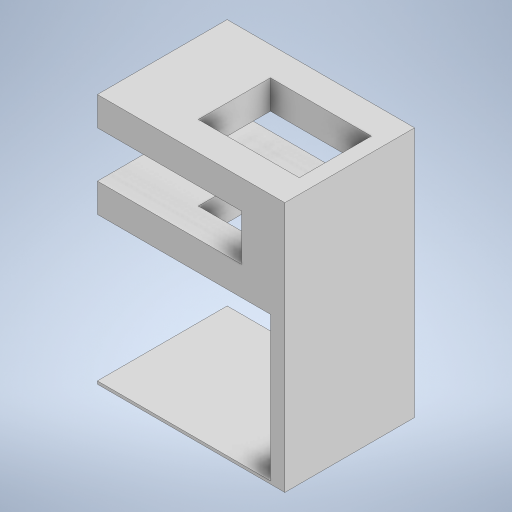
# Autodesk Inventor part: Стенка
Saved by Autodesk Inventor 2023 (Build 270158000, 158)
## iProperties
Created: 2022-04-28
Part Number: Стенка
Material: Типовые
Document SubType Name: Modeling
Designer: User
Density: 1 g/cm^3
Appearance: По умолчанию
Author: User
Autodesk Inventor part; units mm, degrees
ref_plane "YZ Plane" through (0, 0, 0) normal (1, 0, 0) x (0, 1, 0)
ref_plane "XZ Plane" through (0, 0, 0) normal (0, 1, 0) x (-1, 0, 0)
ref_plane "XY Plane" through (0, 0, 0) normal (0, 0, 1) x (1, 0, 0)
sketch "Эскиз1" plane through (0, 0, 0) normal (0, 1, 0) x (-1, 0, 0)
  line L0 (0, 0) -> (60, 0)
  line L1 (60, 0) -> (60, -45)
  line L2 (60, -45) -> (0, -45)
  line L3 (0, -45) -> (0, 0)
  line L4 (0, -22.5) -> (0, 0)
  line L5 (0, 0) -> (0, -10)
  line L6 (0, -10) -> (35, -10)
  line L7 (35, -10) -> (35, -35)
  line L8 (35, -35) -> (0, -35)
  line L9 (35, -22.5) -> (45, -22.5)
  dimension "d0" = 60
  dimension "d1" = 45
  dimension "d3" = 10
  dimension "d4" = 35
  dimension "d5" = 25
  dimension "d6" = 10
  constraints: 20 end point, 4 perpendicular, 2 horizontal, 2 midpoint, 2 parallel, 2 point on line, 1 collinear
  measures "d0" distance of L1.end L2.end
  measures "d1" distance of L0.end L1.end
  measures "d3" distance of L0.start L5.end
  measures "d4" distance of L5.end L6.end
  measures "d5" distance of L6.end L7.end
  measures "d6" distance of L9.start L9.end
extrude "Выдавливание1" add sketch "Эскиз1" along normal blind 10 contours L0 L1 L2 L3 L8 L7 L6
sketch "Эскиз3" plane through (0, 0, -35) normal (1, 0, 0) x (0, 0, -1)
  line L0 (10, 10) -> (-35, 10) projected
  line L1 (10, 10) -> (-35, 10)
  line L2 (-35, 10) -> (-35, -26)
  line L3 (-35, -26) -> (10, -26)
  line L4 (10, -26) -> (10, 10)
  point P0 (-35, 0)
  dimension "d13" = 45
  dimension "d14" = 36
  constraints: 8 end point, 2 parallel, 1 horizontal, 1 perpendicular
  measures "d13" distance of L3.end L2.end
  measures "d14" distance of L2.end L1.end
extrude "Выдавливание3" add sketch "Эскиз3" along normal blind 5
sketch "Эскиз4" plane through (0, -26, -45) normal (0, -1, 0) x (1, 0, 0)
  line L0 (-60, 0) -> (0, 0)
  line L1 (0, 0) -> (0, 45)
  line L2 (0, 45) -> (-60, 45)
  line L3 (-60, 45) -> (-60, 0)
  line L4 (0, 35) -> (-35, 35) projected
  line L5 (-35, 10) -> (0, 10)
  line L6 (0, 10) -> (0, 35)
  line L7 (0, 35) -> (-35, 35)
  line L8 (-35, 35) -> (-35, 10)
  constraints: 16 end point, 4 parallel, 2 horizontal, 2 perpendicular
extrude "Выдавливание4" add sketch "Эскиз4" against normal blind 10 contours L3 L2 L1 L4 L8 L5 L0
sketch "Эскиз5" plane through (0, 0, 0) normal (0, -1, 0) x (1, 0, 0)
  line L0 (-35, -10) -> (-35, -35) projected
  line L1 (-35, -22.5) -> (-45, -22.5)
  circle A0 centre (-45, -22.5) radius 5
  point P0 (0, 0)
  dimension "d19" = 10
  dimension "d20" = 10
  constraints: 2 end point, 1 centre point, 1 coincident, 1 horizontal, 1 midpoint
  measures "d19" distance of L1.start L1.end
  measures "d20" diameter of A0
extrude "Выдавливание5" cut sketch "Эскиз5" along normal blind 24 and the other way blind 6
sketch "Эскиз6" plane through (5, -26, -45) normal (0, -1, 0) x (1, 0, 0)
  line L0 (0, 0) -> (0, 45) projected
  line L1 (-65, 0) -> (0, 0) projected
  line L2 (0, 45) -> (-5, 45)
  line L3 (-5, 45) -> (-5, 0)
  line L4 (-5, 0) -> (0, 0)
  line L5 (0, 0) -> (0, 45)
  constraints: 8 end point, 2 parallel, 1 horizontal, 1 perpendicular, 1 point on line
extrude "Выдавливание6" add sketch "Эскиз6" along normal blind 50
sketch "Эскиз7" plane through (5, -76, -45) normal (0, -1, 0) x (1, 0, 0)
  line L0 (-65, 45) -> (0, 45) projected
  line L1 (0, 45) -> (-65, 45)
  line L2 (-65, 45) -> (-65, 0)
  line L3 (-65, 0) -> (0, 0)
  line L4 (0, 0) -> (0, 45)
  line L5 (-5, 10) -> (-5, 35) projected
  line L6 (-5, 22.5) -> (-15, 22.5)
  line L7 (-15, 22.5) -> (-17.5, 22.5)
  circle A0 centre (-17.5, 22.5) radius 2.5
  point P0 (-5, 45)
  dimension "d27" = 10
  dimension "d28" = 2.5
  constraints: 12 end point, 2 horizontal, 2 parallel, 1 coincident, 1 horizontal alignment, 1 midpoint, 1 perpendicular, 1 point on line, 2 other
  measures "d27" distance of L6.start L6.end
  measures "d28" distance of L6.end L7.end
extrude "Выдавливание7" add sketch "Эскиз7" along normal blind 1
sketch "Эскиз8" plane through (0, 0, -35) normal (-1, 0, 0) x (0, 0, 1)
  line L0 (0, 0) -> (-10, 0) projected
  line L1 (-10, -16) -> (35, -16) projected
  line L2 (-10, 0) -> (0, 0)
  line L3 (0, 0) -> (0, -16)
  line L4 (0, -16) -> (-10, -16)
  line L5 (-10, -16) -> (-10, 0)
  line L6 (35, 0) -> (35, 10) projected
  line L7 (25, -16) -> (35, -16) projected
  line L8 (35, 0) -> (25, 0)
  line L9 (25, 0) -> (25, -16)
  line L10 (25, -16) -> (35, -16)
  line L11 (35, -16) -> (35, 0)
  dimension "d31" = 10
  constraints: 16 end point, 4 parallel, 2 horizontal, 2 perpendicular, 1 point on line
  measures "d31" distance of L3.end L4.end
extrude "Выдавливание8" add sketch "Эскиз8" along normal blind 10
